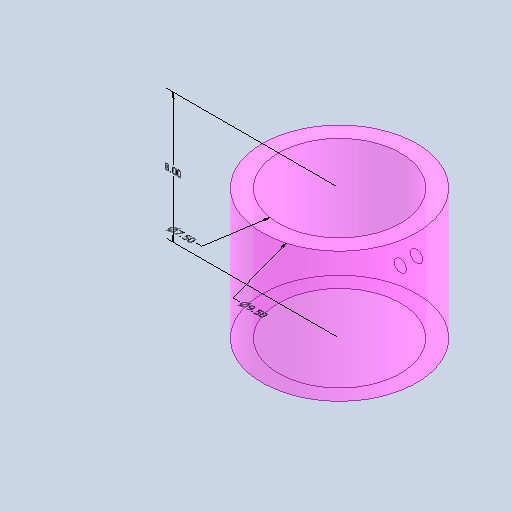
# Autodesk Inventor part: IL-01
Saved by Autodesk Inventor 2022 (Build 260153000, 153)
## iProperties
Company: El Camino College
Created: 2023-05-15
Part Number: IL-01
Material: Fiberglass Insulation
Document SubType Name: Modeling
Designer: Edgar Tejada
Density: 0.0849773 g/cm^3
Appearance: Fiberglass
Mass: 296.868 g
Surface Area: 3110.54 cm^2
Volume: 3493.49 cm^3
Project: Hexagonal Hive
Description: Fiberglass Insulation Layer
Author: Edgar Tejada
Title: Insulation Layer
Subject: Hexagonal Hive
Autodesk Inventor part; units mm, degrees
ref_plane "YZ Plane" through (0, 0, 0) normal (1, 0, 0) x (0, 1, 0)
ref_plane "XZ Plane" through (0, 0, 0) normal (0, 1, 0) x (-1, 0, 0)
ref_plane "XY Plane" through (0, 0, 0) normal (0, 0, 1) x (1, 0, 0)
sketch "Sketch1" plane through (0, 0, 0) normal (0, 1, 0) x (-1, 0, 0)
  circle A0 centre (0, 0) radius 95.25
  circle A1 centre (0, 0) radius 120.65
  dimension "d0" = 190.5
  dimension "d1" = 25.4
  constraints: 2 centre point, 2 coincident
  measures "d0" diameter of A0
  measures "d1" radial gap between concentric circles of A0 A1
extrude "Extrusion1" add sketch "Sketch1" along normal blind 203.2
sketch "Sketch2" plane through (0, 0, 0) normal (0, 0, 1) x (1, 0, 0)
  circle A0 centre (0, 50.8) radius 9.525
  line L0 (120.65, 0) -> (-120.65, 0) projected
  point P0 (0, 0)
  point P1 (0, 0)
  dimension "d5" = 19.05
  dimension "d6" = 50.8
  constraints: 1 centre point, 1 midpoint, 1 vertical alignment
  measures "d5" diameter of A0
  measures "d6" distance of point (0, 0) A0.centre
extrude "Extrusion2" cut sketch "Sketch2" against normal through all
body "Solid1"
